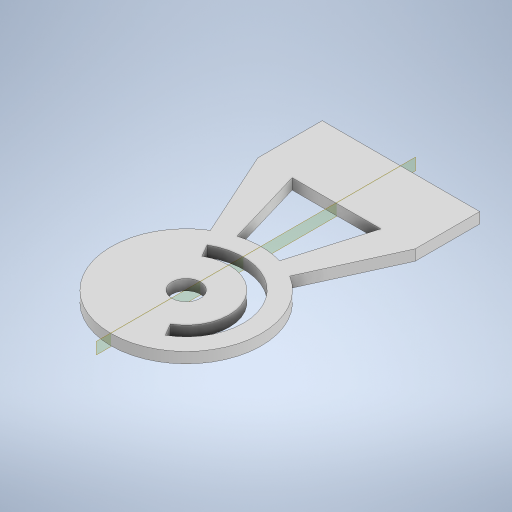
# Autodesk Inventor part: V3_O2
Saved by Autodesk Inventor 2024 (Build 280153000, 153)
## iProperties
Created: 2023-04-22
Part Number: V3_O2
Material: Generisch
Document SubType Name: Sheet Metal
Designer: marco
Density: 1 g/cm^3
Sheet Metal Rule: Standard_mm
Appearance: Vorgabe
Author: marco
Autodesk Inventor part; units mm, degrees
ref_plane "YZ Plane" through (0, 0, 0) normal (1, 0, 0) x (0, 1, 0)
ref_plane "XZ Plane" through (0, 0, 0) normal (0, 1, 0) x (-1, 0, 0)
ref_plane "XY Plane" through (0, 0, 0) normal (0, 0, 1) x (1, 0, 0)
sketch "Skizze1" plane through (0, 0, 0) normal (0, 1, 0) x (-1, 0, 0)
  arc A0 (15.494, 23.3816) -> (6.506, 23.3816) centre (11, 30) ccw
  circle A1 centre (11, 30) radius 10.5
  circle A2 centre (11, 30) radius 2
  circle A3 centre (11, 30) radius 2
  arc A4 (7.25, 36.4952) -> (14.75, 23.5048) centre (11, 30) ccw
  line L0 (14.75, 23.5048) -> (13.75, 25.2369)
  arc A5 (8, 35.1962) -> (14, 24.8038) centre (11, 30) ccw
  arc A6 (7, 36.9282) -> (15, 23.0718) centre (11, 30) ccw
  line L1 (11, 30) -> (15, 23.0718) construction
  line L2 (11, 30) -> (19, 30) construction
  line L3 (11, 30) -> (7, 36.9282) construction
  line L4 (14, 24.8038) -> (15, 23.0718)
  line L5 (8, 35.1962) -> (7, 36.9282)
  line L6 (0, 4.5) -> (0, 9)
  line L7 (0, 9) -> (0, 0)
  line L8 (22, 0) -> (0, 0)
  line L9 (0, 0) -> (22, 0)
  line L10 (22, 9) -> (16.119, 22)
  line L11 (22, 0) -> (22, 9)
  line L12 (22, 9) -> (16.5361, 21.078)
  line L13 (5.881, 22) -> (0, 9)
  line L14 (0, 9) -> (5.4639, 21.078)
  line L15 (8.7349, 22.3274) -> (4.8005, 9)
  line L16 (8.0271, 19.9297) -> (4.8005, 9)
  line L17 (17.1995, 9) -> (4.8005, 9)
  line L18 (4.8005, 9) -> (17.1995, 9)
  line L19 (17.1995, 9) -> (13.9729, 19.9297)
  line L20 (13.2651, 22.3274) -> (17.1995, 9)
  point P0 (21, 0)
  point P1 (6.506, 23.3816)
  point P2 (7, 36.9282)
  dimension "d0" = 21
  dimension "d1" = 6
  dimension "d2" = 8
  dimension "d3" = 60
  dimension "d4" = 180
  constraints: 42 end point, 13 point on circle, 7 centre point, 5 point on line, 4 coincident, 3 collinear, 2 perpendicular, 1 equal length, 1 horizontal, 1 vertical
  measures "d0" diameter of A1
  measures "d1" radius of A5
  measures "d2" radius of A6
  measures "d3" angle of L1 L2
  measures "d4" angle of L1 L3
extrude "Extrusion1" add sketch "Skizze1" along normal blind 1.5 contours A0 A6 L15 A1 L20 L4 L0 A5 L5 | A6 L20 A1 L15 | L15 L17 L19 A1 L10 L11 L8 L7 L6 L13
ref_plane "Arbeitsebene1" through (-11, 0, 0) normal (-1, 0, 0) x (0, 0, 1)
equation "\"Biegeradius\" = Stärke"
equation "\"BreiteBiegungsfreistellung\" = Stärke"
equation "\"TiefeBiegungsfreistellung\" = 0.5 * Stärke"
equation "\"GrößeEckenfreistellung\" = 4 * Stärke"
equation "\"MinimalRest\" = 2 * Stärke"
equation "\"Übergangsradius\" = Biegeradius"
equation "\"JacobiRadiusGröße\" = Biegeradius"
equation "\"Abstandsgröße\" = Stärke"
equation "\"Stärke\" = 0.5"
